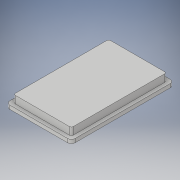
# Autodesk Inventor part: plug
Saved by Autodesk Inventor 2019 (Build 230136000, 136)
## iProperties
Created: 2019-05-30
Part Number: plug
Material: Generic
Document SubType Name: Modeling
Designer: sb002
Density: 1 g/cm^3
Appearance: Default
Author: sb002
## iProperties of the stored document plug_3DPrint.ipt
Created: 2019-05-30
Part Number: plug_3DPrint
Material: Generic
Document SubType Name: Modeling
Designer: sb002
Density: 1 g/cm^3
Appearance: Default
Author: sb002
Autodesk Inventor part; units mm, degrees
ref_plane "YZ Plane" through (0, 0, 0) normal (1, 0, 0) x (0, 1, 0)
ref_plane "XZ Plane" through (0, 0, 0) normal (0, 1, 0) x (-1, 0, 0)
ref_plane "XY Plane" through (0, 0, 0) normal (0, 0, 1) x (1, 0, 0)
sketch "Sketch1" plane through (0, 0, 0) normal (0, 1, 0) x (-1, 0, 0)
  point P0 (0, 0)
sketch "Sketch2" plane through (0, 0, 0) normal (0, 1, 0) x (-1, 0, 0)
  line L0 (4.1714, 6.6076) -> (-13.3286, 6.6076)
  line L1 (-13.3286, 6.6076) -> (-13.3286, -20.8924)
  line L2 (-13.3286, -20.8924) -> (4.1714, -20.8924)
  line L3 (4.1714, -20.8924) -> (4.1714, 6.6076)
  point P0 (0, 0)
  dimension "d0" = 17.5
  dimension "d1" = 27.5
  constraints: 8 end point, 2 parallel, 1 horizontal, 1 perpendicular
  measures "d0" distance of L2.end L1.end
  measures "d1" distance of L1.end L0.end
extrude "Extrusion1" add sketch "Sketch2" along normal blind 1
sketch "Sketch3" plane through (0, 1, 0) normal (0, 1, 0) x (1, 0, 0)
  line L0 (-4.1714, -6.6076) -> (13.3286, -6.6076) projected
  line L1 (-4.1714, -6.6076) -> (-3.1714, -6.6076)
  line L2 (-3.1714, -6.6076) -> (-3.1714, -5.6076)
  line L3 (-3.1714, -5.6076) -> (12.3286, -5.6076)
  line L4 (12.3286, -5.6076) -> (12.3286, 19.8924)
  line L5 (12.3286, 19.8924) -> (-3.1714, 19.8924)
  line L6 (-3.1714, 19.8924) -> (-3.1714, -5.6076)
  point P0 (0, 0)
  dimension "d4" = 1
  dimension "d5" = 1
  dimension "d6" = 15.5
  dimension "d7" = 25.5
  constraints: 12 end point, 2 parallel, 2 perpendicular, 1 horizontal, 1 point on line
  measures "d4" distance of L0.start L1.end
  measures "d5" distance of L1.end L2.end
  measures "d6" distance of L5.end L4.end
  measures "d7" distance of L4.end L3.end
extrude "Extrusion2" add sketch "Sketch3" along normal blind 2
fillet "Fillet1" radius 1 4 edges at (-4.1714, 0.5, -20.8924) (-4.1714, 0.5, 6.6076) (13.3286, 0.5, 6.6076) (13.3286, 0.5, -20.8924)
fillet "Fillet2" radius 0.5 4 edges at (12.3286, 2, -19.8924) (12.3286, 2, 5.6076) (-3.1714, 2, -19.8924) (-3.1714, 2, 5.6076)
body "Solid1"
